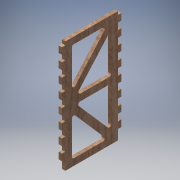
# Autodesk Inventor part: CrossBar2
Saved by Autodesk Inventor 2019 (Build 230136000, 136)
## iProperties
Created: 2019-01-14
Part Number: CrossBar2
Material: Wood (Birch)
Document SubType Name: Modeling
Designer: nxgam
Density: 0.55 g/cm^3
Appearance: Birch - Natural Polished
Author: nxgam
Autodesk Inventor part; units mm, degrees
ref_plane "YZ Plane" through (0, 0, 0) normal (1, 0, 0) x (0, 1, 0)
ref_plane "XZ Plane" through (0, 0, 0) normal (0, 1, 0) x (-1, 0, 0)
ref_plane "XY Plane" through (0, 0, 0) normal (0, 0, 1) x (1, 0, 0)
sketch "Sketch1" plane through (0, 0, 0) normal (1, 0, 0) x (0, 1, 0)
  line L0 (0, 0) -> (81.28, 0)
  line L1 (81.28, 0) -> (81.28, -91.44) construction
  line L2 (81.28, -91.44) -> (0, -91.44)
  line L3 (0, -91.44) -> (0, 0)
  line L4 (0, 0) -> (10.16, 0)
  line L5 (10.16, 0) -> (10.16, -5.08)
  line L6 (10.16, -5.08) -> (0, -5.08)
  line L7 (0, -5.08) -> (0, 0)
  line L8 (20.32, 0) -> (30.48, 0)
  line L9 (30.48, 0) -> (30.48, -5.08)
  line L10 (30.48, -5.08) -> (20.32, -5.08)
  line L11 (20.32, -5.08) -> (20.32, 0)
  line L12 (40.64, 0) -> (50.8, 0)
  line L13 (50.8, 0) -> (50.8, -5.08)
  line L14 (50.8, -5.08) -> (40.64, -5.08)
  line L15 (40.64, -5.08) -> (40.64, 0)
  line L16 (60.96, 0) -> (71.12, 0)
  line L17 (71.12, 0) -> (71.12, -5.08)
  line L18 (71.12, -5.08) -> (60.96, -5.08)
  line L19 (60.96, -5.08) -> (60.96, 0)
  line L20 (81.28, -45.72) -> (0, -45.72) construction
  line L21 (0, -91.44) -> (81.28, -91.44)
  line L22 (0, -91.44) -> (10.16, -91.44)
  line L23 (10.16, -91.44) -> (10.16, -86.36)
  line L24 (10.16, -86.36) -> (0, -86.36)
  line L25 (0, -86.36) -> (0, -91.44)
  line L26 (20.32, -91.44) -> (30.48, -91.44)
  line L27 (30.48, -91.44) -> (30.48, -86.36)
  line L28 (30.48, -86.36) -> (20.32, -86.36)
  line L29 (20.32, -86.36) -> (20.32, -91.44)
  line L30 (40.64, -91.44) -> (50.8, -91.44)
  line L31 (50.8, -91.44) -> (50.8, -86.36)
  line L32 (50.8, -86.36) -> (40.64, -86.36)
  line L33 (40.64, -86.36) -> (40.64, -91.44)
  line L34 (60.96, -91.44) -> (71.12, -91.44)
  line L35 (71.12, -91.44) -> (71.12, -86.36)
  line L36 (71.12, -86.36) -> (60.96, -86.36)
  line L37 (60.96, -86.36) -> (60.96, -91.44)
  line L38 (81.28, -86.36) -> (81.28, -91.44)
  line L39 (0, 0) -> (91.44, 0) construction
  line L40 (0, -91.44) -> (0, 0) construction
  line L41 (81.28, -10.16) -> (0, -10.16) construction
  line L42 (0, -10.16) -> (0, -81.28) construction
  line L43 (0, -81.28) -> (81.28, -81.28) construction
  line L44 (81.28, -81.28) -> (81.28, -10.16) construction
  line L45 (81.28, -10.16) -> (0, -81.28) construction
  line L46 (76.2, -28.3521) -> (76.2, -73.025)
  line L47 (73.025, -76.2) -> (21.9703, -76.2)
  line L48 (19.8795, -70.6356) -> (70.9342, -25.9627)
  arc A0 (76.2, -28.3521) -> (70.9342, -25.9627) centre (73.025, -28.3521) ccw
  arc A1 (73.025, -76.2) -> (76.2, -73.025) centre (73.025, -73.025) ccw
  arc A2 (19.8795, -70.6356) -> (21.9703, -76.2) centre (21.9703, -73.025) ccw
  line L49 (8.255, -15.24) -> (59.3097, -15.24)
  line L50 (61.4005, -20.8044) -> (10.3458, -65.4773)
  line L51 (5.08, -63.0879) -> (5.08, -18.415)
  arc A3 (61.4005, -20.8044) -> (59.3097, -15.24) centre (59.3097, -18.415) ccw
  arc A4 (5.08, -63.0879) -> (10.3458, -65.4773) centre (8.255, -63.0879) ccw
  arc A5 (8.255, -15.24) -> (5.08, -18.415) centre (8.255, -18.415) ccw
  line L52 (81.28, -45.72) -> (162.56, -45.72) construction
  line L53 (81.28, -10.16) -> (162.56, -10.16) construction
  line L54 (162.56, -81.28) -> (81.28, -81.28) construction
  line L55 (81.28, -10.16) -> (162.56, -81.28) construction
  line L56 (86.36, -28.3521) -> (86.36, -73.025)
  line L57 (89.535, -76.2) -> (140.5897, -76.2)
  line L58 (142.6805, -70.6356) -> (91.6258, -25.9627)
  arc A6 (91.6258, -25.9627) -> (86.36, -28.3521) centre (89.535, -28.3521) ccw
  arc A7 (86.36, -73.025) -> (89.535, -76.2) centre (89.535, -73.025) ccw
  arc A8 (140.5897, -76.2) -> (142.6805, -70.6356) centre (140.5897, -73.025) ccw
  line L59 (154.305, -15.24) -> (103.2503, -15.24)
  line L60 (101.1595, -20.8044) -> (152.2142, -65.4773)
  line L61 (157.48, -63.0879) -> (157.48, -18.415)
  arc A9 (103.2503, -15.24) -> (101.1595, -20.8044) centre (103.2503, -18.415) ccw
  arc A10 (152.2142, -65.4773) -> (157.48, -63.0879) centre (154.305, -63.0879) ccw
  arc A11 (157.48, -18.415) -> (154.305, -15.24) centre (154.305, -18.415) ccw
  line L62 (132.08, -86.36) -> (121.92, -86.36)
  line L63 (101.6, -86.36) -> (101.6, -91.44)
  line L64 (101.6, -91.44) -> (111.76, -91.44)
  line L65 (111.76, -91.44) -> (111.76, -86.36)
  line L66 (111.76, -86.36) -> (101.6, -86.36)
  line L67 (91.44, -86.36) -> (81.28, -86.36)
  line L68 (91.44, -91.44) -> (91.44, -86.36)
  line L69 (81.28, -91.44) -> (91.44, -91.44)
  line L70 (81.28, -91.44) -> (162.56, -91.44)
  line L71 (162.56, -91.44) -> (81.28, -91.44)
  line L72 (81.28, -81.28) -> (162.56, -81.28) construction
  line L73 (81.28, -10.16) -> (81.28, -81.28) construction
  line L74 (162.56, 0) -> (162.56, -91.44)
  line L75 (81.28, -91.44) -> (81.28, 0) construction
  line L76 (81.28, -91.44) -> (81.28, 0) construction
  line L77 (81.28, 0) -> (162.56, 0)
  line L78 (81.28, 0) -> (91.44, 0)
  line L79 (91.44, 0) -> (91.44, -5.08)
  line L80 (81.28, -5.08) -> (81.28, 0)
  line L81 (91.44, -5.08) -> (81.28, -5.08)
  line L82 (111.76, -5.08) -> (101.6, -5.08)
  line L83 (101.6, 0) -> (111.76, 0)
  line L84 (101.6, -5.08) -> (101.6, 0)
  line L85 (111.76, 0) -> (111.76, -5.08)
  line L86 (132.08, -5.08) -> (121.92, -5.08)
  line L87 (132.08, 0) -> (132.08, -5.08)
  line L88 (121.92, -5.08) -> (121.92, 0)
  line L89 (121.92, 0) -> (132.08, 0)
  line L90 (142.24, -5.08) -> (142.24, 0)
  line L91 (152.4, -5.08) -> (142.24, -5.08)
  line L92 (142.24, 0) -> (152.4, 0)
  line L93 (152.4, 0) -> (152.4, -5.08)
  line L94 (81.28, -86.36) -> (81.28, -91.44)
  line L95 (152.4, -86.36) -> (142.24, -86.36)
  line L96 (142.24, -91.44) -> (152.4, -91.44)
  line L97 (162.56, -86.36) -> (162.56, -91.44)
  line L98 (132.08, -91.44) -> (132.08, -86.36)
  line L99 (81.28, 0) -> (172.72, 0) construction
  line L100 (152.4, -91.44) -> (152.4, -86.36)
  line L101 (121.92, -86.36) -> (121.92, -91.44)
  line L102 (142.24, -86.36) -> (142.24, -91.44)
  line L103 (162.56, -81.28) -> (162.56, -10.16) construction
  line L104 (121.92, -91.44) -> (132.08, -91.44)
  line L105 (162.56, -10.16) -> (81.28, -10.16) construction
  line L106 (243.84, -81.28) -> (162.56, -81.28) construction
  line L107 (162.56, -45.72) -> (243.84, -45.72) construction
  line L108 (162.56, -10.16) -> (243.84, -81.28) construction
  line L109 (162.56, -10.16) -> (243.84, -10.16) construction
  line L110 (162.56, 0) -> (0, 0)
  line L111 (0, 0) -> (0, -91.44)
  line L112 (0, -91.44) -> (162.56, -91.44)
  line L113 (162.56, -91.44) -> (162.56, 0)
  point P0 (40.64, -45.72)
  point P1 (121.92, -45.72)
  point P2 (81.28, -45.72)
  point P3 (203.2, -45.72)
  dimension "d0" = 81.28
  dimension "d1" = 91.44
  dimension "d2" = 10.16
  dimension "d3" = 5.08
  dimension "d6" = 20.32
  dimension "d12" = 5.08
  dimension "d13" = 0
  dimension "d14" = 3.175
  dimension "d15" = 3.175
  dimension "d16" = 10.16
  dimension "d17" = 10.16
  dimension "d18" = 5.08
  dimension "d20" = 10.16
  dimension "d21" = 5.08
  dimension "d26" = 81.28
  constraints: 228 end point, 38 symmetric about line, 24 point on circle, 12 centre point, 12 tangent, 10 parallel, 7 horizontal, 5 midpoint, 5 perpendicular, 4 equal radius, 1 coincident, 1 collinear, 1 point on line, 129 other
  measures "d0" distance of L1.end L2.end
  measures "d1" distance of L0.end L1.end
  measures "d2" distance of L5.end L6.end
  measures "d3" distance of L4.end L5.end
  measures "d6" distance of L0.start L8.start
  measures "d12" distance between parallel lines of L28 L43
  measures "d13" distance between parallel lines of L44 L1
  measures "d14" radius of A0
  measures "d15" radius of A3
  measures "d16" distance between parallel lines of L50 L48
  measures "d17" distance between parallel lines of L28 L47
  measures "d18" distance between parallel lines of L3 L51
  measures "d20" distance between parallel lines of L14 L49
  measures "d21" distance between parallel lines of L1 L46
  measures "d26" distance of L32.start L62.start
extrude "Extrusion2" add sketch "Sketch1" along normal blind 5.08 contours L0 L11 L10 L9 L15 L14 L13 L19 L18 L17 L80 L81 L79 L77 L84 L82 L85 L88 L86 L87 L90 L91 L93 L74 L70 L100 L95 L102 L98 L62 L101 L65 L66 L63 L68 L67 L38 L2 L35 L36 L37 L31 L32 L33 L27 L28 L29 L23 L24 L3 L6 L5
sketch "Sketch2" plane through (0, 162.56, 0) normal (0, 1, 0) x (1, 0, 0)
  line L0 (0, 91.44) -> (0, 0) projected
  line L1 (0, 0) -> (5.08, 0) projected
  line L2 (5.08, 91.44) -> (5.08, 0) projected
  line L3 (0, 91.44) -> (5.08, 91.44) projected
  line L4 (0, 5.08) -> (0, 0) projected
  line L5 (5.08, 5.08) -> (5.08, 86.36) projected
  line L6 (0, 5.08) -> (5.08, 5.08)
  line L7 (5.08, 5.08) -> (5.08, 86.36)
  line L8 (5.08, 86.36) -> (0, 86.36)
  line L9 (0, 86.36) -> (0, 5.08)
  constraints: 8 end point, 2 parallel, 1 horizontal, 1 perpendicular
extrude "Extrusion3" add sketch "Sketch2" along normal blind 5.08 contours L8 L2 L6 L0
thicken "Thicken1" operation add thickness 5.08 both sides no extend neighbours yes toward (0, -1, 0) faces at (1.6933, 0, -32.1733)
equation "\"d16\" = d17"
equation "\"d18\" = d21"
equation "\"d20\" = d17"
equation "\"d26\" = d0"
body "Solid2"
